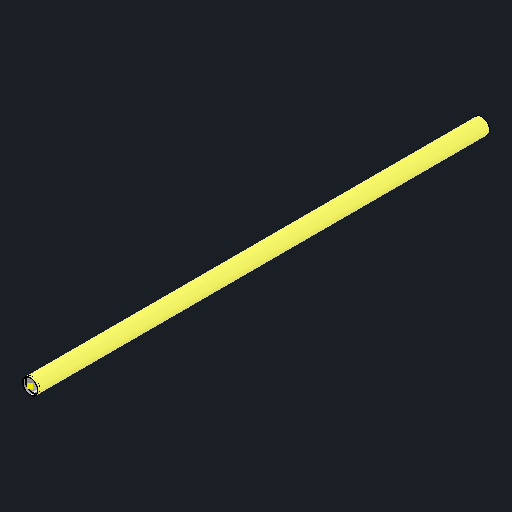
# Autodesk Inventor part: B_probe_pipe_5_for-non-bellows_1
Saved by Autodesk Inventor 2027.1 (Build 311270010, 270A)
## iProperties
Created: 2026-07-09
Part Number: B_probe_pipe_5_for-non-bellows_1
Material: ステンレス鋼
Document SubType Name: Modeling
Designer: zetsu
Density: 8 g/cm^3
Appearance: 半つや出し
Author: zetsu
Autodesk Inventor part; units mm, degrees
ref_plane "YZ Plane" through (0, 0, 0) normal (1, 0, 0) x (0, 1, 0)
ref_plane "XZ Plane" through (0, 0, 0) normal (0, 1, 0) x (-1, 0, 0)
ref_plane "XY Plane" through (0, 0, 0) normal (0, 0, 1) x (1, 0, 0)
sketch "スケッチ1" plane through (0, 0, 0) normal (0, 0, 1) x (1, 0, 0)
  circle A0 centre (0, 0) radius 17
  circle A1 centre (0, 0) radius 14.2
  dimension "d0" = 34
  dimension "d1" = 28.4
  constraints: 2 centre point, 2 coincident
  measures "d0" diameter of A0
  measures "d1" diameter of A1
extrude "押し出し1" add sketch "スケッチ1" along normal blind 1000
sketch "スケッチ2" plane through (0, 0, 1000) normal (0, 0, 1) x (1, 0, 0)
  point P0 (0, 0)
sketch "スケッチ3" plane through (0, 0, 1000) normal (0, 0, 1) x (1, 0, 0)
  circle A0 centre (0, 0) radius 16
  dimension "d4" = 32
  constraints: 1 centre point, 1 coincident
  measures "d4" diameter of A0
extrude "押し出し2" cut sketch "スケッチ3" against normal blind 5
